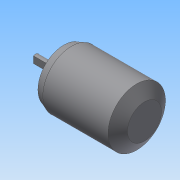
# Autodesk Inventor part: motor
Saved by Autodesk Inventor 2015 (Build 190159000, 159)
## iProperties
Created: 2016-01-05
Part Number: motor
Material: Generic
Document SubType Name: Modeling
Designer: JoshuaYuan
Density: 1 g/cm^3
Appearance: Default
Author: JoshuaYuan
Autodesk Inventor part; units mm, degrees
ref_plane "YZ Plane" through (0, 0, 0) normal (1, 0, 0) x (0, 1, 0)
ref_plane "XZ Plane" through (0, 0, 0) normal (0, 1, 0) x (-1, 0, 0)
ref_plane "XY Plane" through (0, 0, 0) normal (0, 0, 1) x (1, 0, 0)
sketch "Sketch1" plane through (0, 0, 0) normal (0, 0, 1) x (1, 0, 0)
  line L0 (0, 0) -> (0, -4)
  line L1 (0, -4) -> (29, -4)
  line L2 (29, -4) -> (29, -26.5)
  line L3 (29, -26.5) -> (37, -29.5)
  line L4 (37, -29.5) -> (104, -29.5)
  line L5 (104, -29.5) -> (112, -17.5)
  line L6 (112, -17.5) -> (112, 0)
  line L7 (-22.4, 0) -> (134.4, 0) projected
  line L8 (0, -35.4) -> (0, 5.9) projected
  line L9 (112, 0) -> (0, 0)
  dimension "d7" = 22.5
  dimension "d9" = 8
  dimension "d10" = 67
  dimension "d14" = 4
  dimension "d15" = 112
  dimension "d16" = 29.5
  dimension "d17" = 17.5
  dimension "d18" = 29
  constraints: 17 end point, 2 horizontal, 2 perpendicular, 1 collinear, 1 parallel, 1 vertical, 1 other
  measures "d7" distance of L1.end L2.end
  measures "d9" distance from line of L3.end L2
  measures "d10" distance of L3.end L4.end
  measures "d14" distance of L0.start L0.end
  measures "d15" distance of L0.start L6.end
  measures "d16" distance between parallel lines of L9 L4
  measures "d17" distance of L5.end L6.end
  measures "d18" distance of L0.end L1.end
revolve "motor body" add sketch "Sketch1" angle 360 about axis through (-10, 0, 0) along (1, 0, 0)
sketch "Sketch4" plane through (0, 0, 0) normal (-1, 0, 0) x (0, 0, 1)
  circle A0 centre (0, 0) radius 4
  circle A1 centre (0, 0) radius 4 projected
  line L0 (2.0699, 3.4228) -> (2.0699, -3.4228)
  line L1 (0, -41.3) -> (0, 41.3) projected
  constraints: 4 point on circle, 2 end point, 1 centre point, 1 coincident, 1 parallel
extrude "axis slot" cut sketch "Sketch4" against normal blind 25 contours A0 L0
sketch "Sketch5" plane through (29, 0, 0) normal (-1, 0, 0) x (0, 0, 1)
  circle A0 centre (15.5, 15.5) radius 1.5875
  line L0 (0, -41.3) -> (0, 41.3) projected
  line L1 (-41.3, 0) -> (41.3, 0) projected
  circle A1 centre (15.5, -15.5) radius 1.5875
  circle A2 centre (-15.5, 15.5) radius 1.5875
  circle A3 centre (-15.5, -15.5) radius 1.5875
  point P0 (0, 0)
  dimension "d22" = 3.175
  dimension "d25" = 31
  dimension "d28" = 31
  dimension "d31" = 15.5
  dimension "d32" = 15.5
  constraints: 4 centre point, 1 horizontal, 1 vertical, 6 other
  measures "d22" diameter of A0
  measures "d25" distance of A0.centre A1.centre
  measures "d28" distance of A0.centre A2.centre
  measures "d31" horizontal distance of point (0, 0) A0.centre
  measures "d32" horizontal distance of point (0, 0) A0.centre
extrude "mounting holes" cut sketch "Sketch5" against normal blind 4
ref_plane "Work Plane1" through (70.5, 0, -29.5) normal (0, 0, 1) x (1, 0, 0)
sketch "Sketch6" plane through (70.5, 0, -29.5) normal (0, 0, 1) x (1, 0, 0)
  line L0 (-37.75, 10) -> (-37.75, -10) construction
  line L1 (-40.5, 10) -> (-40.5, -10)
  line L2 (-35, -10) -> (-35, 10)
  arc A0 (-35, 10) -> (-40.5, 10) centre (-37.75, 10) ccw
  arc A1 (-40.5, -10) -> (-35, -10) centre (-37.75, -10) ccw
  line L3 (-41.5, 26.5) -> (-41.5, -26.5) projected
  line L4 (-33.5, 29.5) -> (-33.5, -29.5) projected
  line L5 (-92.9, 0) -> (63.9, 0) projected
  point P0 (-70.5, 0)
  point P1 (-37.75, 0)
  dimension "d35" = 20
  dimension "d36" = 5.5
  dimension "d37" = 1.5
  constraints: 8 end point, 4 point on circle, 4 tangent, 2 centre point, 1 midpoint, 1 parallel, 1 point on line, 1 vertical
  measures "d35" distance of L0.end L0.start
  measures "d36" distance between parallel lines of L1 L2
  measures "d37" distance between parallel lines of L2 L4
extrude "cable hole" cut sketch "Sketch6" along normal blind 10
body "Solid2"
